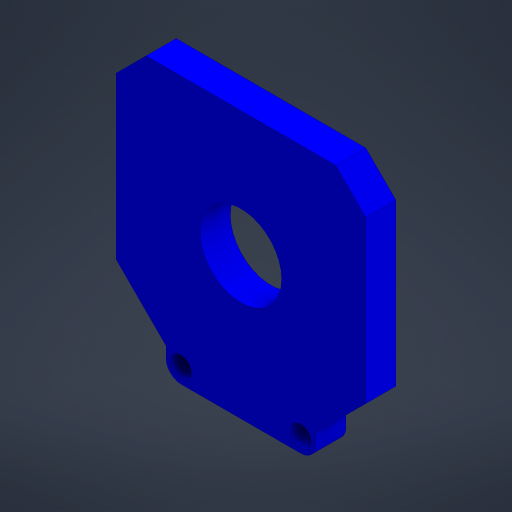
# Autodesk Inventor part: Filter Mount (SM1)
Saved by Autodesk Inventor 2023.4 (Build 274418000, 418)
## iProperties
Created: 2022-11-16
Part Number: Filter Mount (SM1)
Material: Generic
Document SubType Name: Modeling
Designer: xSibe
Density: 1 g/cm^3
Appearance: Plastic Blue
Author: xSibe
Autodesk Inventor part; units mm, degrees
ref_plane "YZ Plane" through (0, 0, 0) normal (1, 0, 0) x (0, 1, 0)
ref_plane "XZ Plane" through (0, 0, 0) normal (0, 1, 0) x (-1, 0, 0)
ref_plane "XY Plane" through (0, 0, 0) normal (0, 0, 1) x (1, 0, 0)
sketch "Sketch1" plane through (0, 0, 0) normal (0, 0, 1) x (1, 0, 0)
  line L0 (22.9, 0.025) -> (-22.9, 0.025) projected
  line L1 (22.9, 42.1) -> (22.9, 0.025) projected
  line L2 (22.9, 42.1) -> (17.05, 42.1) projected
  line L3 (17.05, 7.7) -> (17.05, 42.1) projected
  line L4 (-17.05, 7.7) -> (17.05, 7.7) projected
  line L5 (-17.05, 7.7) -> (-17.05, 42.1) projected
  line L6 (-17.05, 42.1) -> (-22.9, 42.1) projected
  line L7 (-22.9, 0.025) -> (-22.9, 42.1) projected
  circle A0 centre (19.9, 34.8) radius 2.0625 projected
  circle A1 centre (-19.9, 34.8) radius 2.0625 projected
  circle A2 centre (19.9, 15) radius 2.0625 projected
  circle A3 centre (-19.9, 15) radius 2.0625 projected
  circle A4 centre (10, 3.85) radius 1.5625 projected
  circle A5 centre (-10, 3.85) radius 1.5625 projected
  line L8 (-10, 3.85) -> (10, 3.85) construction
  line L9 (-10, 1.35) -> (10, 1.35)
  line L10 (10, 6.35) -> (-10, 6.35)
  arc A6 (-10, 6.35) -> (-10, 1.35) centre (-10, 3.85) ccw
  arc A7 (10, 1.35) -> (10, 6.35) centre (10, 3.85) ccw
  line L11 (-12.5, 3.85) -> (12.5, 3.85)
  line L12 (12.5, 3.85) -> (12.5, 7.7)
  line L13 (12.5, 7.7) -> (-12.5, 7.7)
  line L14 (-12.5, 7.7) -> (-12.5, 3.85)
  line L15 (-17.05, 42.1) -> (17.05, 42.1)
  line L16 (17.05, 42.1) -> (17.05, 7.7)
  line L17 (17.05, 7.7) -> (-17.05, 7.7)
  line L18 (-17.05, 7.7) -> (-17.05, 42.1)
  line L19 (15.8, 45.85) -> (-15.8, 45.85)
  line L20 (-20.8, 40.85) -> (-20.8, 13.95)
  line L21 (-10.8, 3.95) -> (10.8, 3.95)
  line L22 (20.8, 13.95) -> (20.8, 40.85)
  line L23 (-20.8, 40.85) -> (-15.8, 45.85)
  line L24 (15.8, 45.85) -> (20.8, 40.85)
  line L25 (-20.8, 13.95) -> (-10.8, 3.95)
  line L26 (10.8, 3.95) -> (20.8, 13.95)
  line L27 (-17.05, 24.9) -> (17.05, 24.9)
  circle A8 centre (0, 24.9) radius 6.7838
  circle A9 centre (-10, 3.85) radius 1.7188
  circle A10 centre (10, 3.85) radius 1.7188
  point P0 (0, 0)
  point P1 (0, 3.85)
  point P2 (20.8, 45.85)
  point P3 (-20.8, 45.85)
  point P4 (-20.8, 3.95)
  point P5 (20.8, 3.95)
  point P6 (-12.0828, 5.2328)
  point P7 (12.0828, 5.2328)
  point P8 (12.5, 5.65)
  point P9 (-12.5, 5.65)
  dimension "d0" = 5
  dimension "d1" = 25
  dimension "d2" = 3.75
  dimension "d3" = 5
  dimension "d4" = 5
  dimension "d5" = 5
  dimension "d6" = 5
  dimension "d7" = 10
  dimension "d8" = 10
  dimension "d9" = 10
  dimension "d10" = 10
  dimension "d11" = 13.5675
  dimension "d14" = 0.1562
  dimension "d15" = 0.1562
  constraints: 42 end point, 9 point on line, 7 parallel, 5 centre point, 5 point on circle, 4 midpoint, 4 tangent, 3 horizontal, 3 perpendicular, 3 other
  measures "d0" diameter of A7
  measures "d1" distance of L13.end L12.end
  measures "d2" distance between parallel lines of L15 L19
  measures "d3" distance of L20.start point (-20.8, 45.85)
  measures "d4" distance of L19.end point (-20.8, 45.85)
  measures "d5" distance of L19.start point (20.8, 45.85)
  measures "d6" distance of L22.end point (20.8, 45.85)
  measures "d7" distance of L20.end point (-20.8, 3.95)
  measures "d8" distance of L21.start point (-20.8, 3.95)
  measures "d9" distance of L21.end point (20.8, 3.95)
  measures "d10" distance of L22.start point (20.8, 3.95)
  measures "d11" diameter of A8
  measures "d14" radial gap between concentric circles of A5 A9
  measures "d15" radial gap between concentric circles of A4 A10
extrude "Extrusion1" add sketch "Sketch1" along normal mid plane 5 contours L24 L22 A0 A2 L26 L3 L2 | L2 L15 L6 L23 L19 L24 | L6 L5 L25 A3 L20 A1 L23 | L3 L27 A8 L5 L15 | L3 L26 L4 L25 L5 L27 A8 | L22 A0 | A1 L20 | L26 L12 L4 | A2 L22 L26 | L25 L20 A3 | L4 L14 L25 | L12 L26 A7 L10 A6 L25 L14 L4 | L12 A7 L26 | L25 A6 L14 | L11 A10 L26 A7 | A7 L9 A6 L11 A9 A10 | L26 A10 L21 A9 L25 A6 L10 A7 | A6 L25 A9 L11 | L11 A9 L21 A10 picked at (19.8174, 34.7184) picked at (-19.8298, 34.6468) picked at (19.4173, 15.7688) picked at (-19.2349, 15.6172)
equation "\"d4\" = d3"
equation "\"d5\" = d3"
equation "\"d6\" = d5"
equation "\"d8\" = d7"
equation "\"d9\" = d7"
equation "\"d10\" = d9"
body "Solid1"
